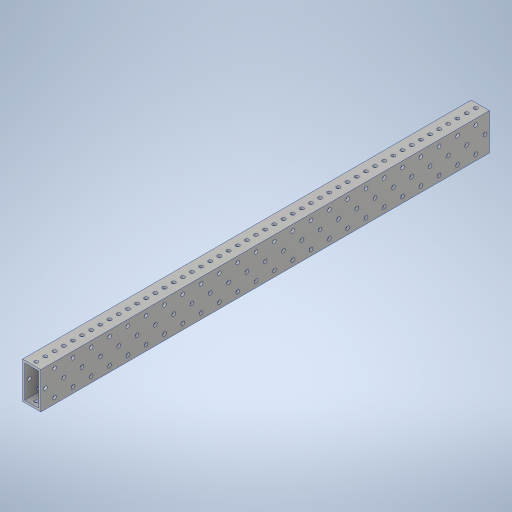
# Autodesk Inventor part: DB1-002
Saved by Autodesk Inventor 2023.4 (Build 274418000, 418)
## iProperties
Created: 2025-01-09
Part Number: DB1-002
Material: Aluminum 6061
Document SubType Name: Modeling
Designer: mavericks
Mass: 304.185 g
Surface Area: 718.547 cm^2
Volume: 112.661 cm^3
Density: 2.7 g/cm^3
Appearance: Aluminum - Flat
RuleStatus: InUse
AfterDocNew0: SHOW
AfterDocOpen0: SHOW
Author: mavericks
Autodesk Inventor part; units mm, degrees
ref_plane "YZ Plane" through (0, 0, 0) normal (1, 0, 0) x (0, 1, 0)
ref_plane "XZ Plane" through (0, 0, 0) normal (0, 1, 0) x (-1, 0, 0)
ref_plane "XY Plane" through (0, 0, 0) normal (0, 0, 1) x (1, 0, 0)
sketch "Sketch1" plane through (0, 0, 0) normal (0, 0, 1) x (1, 0, 0)
  line L0 (-12.7, -25.4) -> (12.7, -25.4)
  line L1 (12.7, -25.4) -> (12.7, 25.4)
  line L2 (12.7, 25.4) -> (-12.7, 25.4)
  line L3 (-12.7, 25.4) -> (-12.7, -25.4)
  line L4 (-12.7, -25.4) -> (12.7, 25.4) construction
  line L5 (12.7, -25.4) -> (-12.7, 25.4) construction
  line L6 (-9.525, 22.225) -> (9.525, 22.225)
  line L7 (9.525, 22.225) -> (9.525, -22.225)
  line L8 (9.525, -22.225) -> (-9.525, -22.225)
  line L9 (-9.525, -22.225) -> (-9.525, 22.225)
  point P0 (0, 0)
  dimension "width" = 25.4
  dimension "height" = 50.8
  dimension "thickness" = 3.175
  constraints: 20 end point, 4 parallel, 2 midpoint, 2 perpendicular, 1 horizontal, 3 other
  measures "width" distance of L2.end L1.end
  measures "height" distance of L1.end L0.end
  measures "thickness" distance between parallel lines of L2 L6
extrude "Extrusion1" add sketch "Sketch1" along normal mid plane 622.3
sketch "Sketch2" plane through (-12.7, 25.4, 311.15) normal (0, 1, 0) x (1, 0, 0)
  line L0 (12.7, 323.85) -> (12.7, 298.45) construction
  line L1 (0, 622.3) -> (0, 0) construction
  point P0 (12.7, 311.15)
  point P1 (12.7, 311.15)
  point P2 (12.7, 285.75)
  point P3 (12.7, 273.05)
  point P4 (12.7, 260.35)
  point P5 (12.7, 247.65)
  point P6 (12.7, 234.95)
  point P7 (12.7, 222.25)
  point P8 (12.7, 209.55)
  point P9 (12.7, 196.85)
  point P10 (12.7, 184.15)
  point P11 (12.7, 171.45)
  point P12 (12.7, 158.75)
  point P13 (12.7, 146.05)
  point P14 (12.7, 133.35)
  point P15 (12.7, 120.65)
  point P16 (12.7, 107.95)
  point P17 (12.7, 95.25)
  point P18 (12.7, 82.55)
  point P19 (12.7, 69.85)
  point P20 (12.7, 57.15)
  point P21 (12.7, 44.45)
  point P22 (12.7, 31.75)
  point P23 (12.7, 19.05)
  point P24 (12.7, 6.35)
  point P25 (12.7, 336.55)
  point P26 (12.7, 349.25)
  point P27 (12.7, 361.95)
  point P28 (12.7, 374.65)
  point P29 (12.7, 387.35)
  point P30 (12.7, 400.05)
  point P31 (12.7, 412.75)
  point P32 (12.7, 425.45)
  point P33 (12.7, 438.15)
  point P34 (12.7, 450.85)
  point P35 (12.7, 463.55)
  point P36 (12.7, 476.25)
  point P37 (12.7, 488.95)
  point P38 (12.7, 501.65)
  point P39 (12.7, 514.35)
  point P40 (12.7, 527.05)
  point P41 (12.7, 539.75)
  point P42 (12.7, 552.45)
  point P43 (12.7, 565.15)
  point P44 (12.7, 577.85)
  point P45 (12.7, 590.55)
  point P46 (12.7, 603.25)
  point P47 (12.7, 615.95)
  point P48 (12.7, 311.15)
  dimension "d6" = 25.4
  dimension "d9" = 12.7
  dimension "d16" = 12.7
  constraints: 3 vertical, 2 coincident, 2 end point, 2 vertical alignment, 1 midpoint, 46 other
  measures "d6" distance of L0.start L0.end
  measures "d9" distance of L0.end point (12.7, 285.75)
  measures "d16" distance of L0.start point (12.7, 336.55)
hole "Hole1" at (0, 25.4, 12.7) at (0, 25.4, -12.7) at (0, 25.4, 25.4) at (0, 25.4, 38.1) at (0, 25.4, 50.8) at (0, 25.4, 63.5) at (0, 25.4, 76.2) at (0, 25.4, 88.9) at (0, 25.4, 101.6) at (0, 25.4, 114.3) at (0, 25.4, 127) at (0, 25.4, 139.7) at (0, 25.4, 152.4) at (0, 25.4, 165.1) at (0, 25.4, 177.8) at (0, 25.4, 190.5) at (0, 25.4, 203.2) at (0, 25.4, 215.9) at (0, 25.4, 228.6) at (0, 25.4, 241.3) at (0, 25.4, 254) at (0, 25.4, 266.7) at (0, 25.4, 279.4) at (0, 25.4, 292.1) at (0, 25.4, 304.8) at (0, 25.4, -25.4) at (0, 25.4, -38.1) at (0, 25.4, -50.8) at (0, 25.4, -63.5) at (0, 25.4, -76.2) at (0, 25.4, -88.9) at (0, 25.4, -101.6) at (0, 25.4, -114.3) at (0, 25.4, -127) at (0, 25.4, -139.7) at (0, 25.4, -152.4) at (0, 25.4, -165.1) at (0, 25.4, -177.8) at (0, 25.4, -190.5) at (0, 25.4, -203.2) at (0, 25.4, -215.9) at (0, 25.4, -228.6) at (0, 25.4, -241.3) at (0, 25.4, -254) at (0, 25.4, -266.7) at (0, 25.4, -279.4) at (0, 25.4, -292.1) at (0, 25.4, -304.8) at (0, 25.4, 0) direction (0, -1, 0) diameter 5.1054 end through all clearance for "Flat Head Machine Screw (82)" size "#10" standard "Ansi Unified Screw Threads"
sketch "Sketch3" plane through (12.7, -25.4, 311.15) normal (1, 0, 0) x (0, 0, -1)
  line L0 (298.45, 42.8625) -> (298.45, 7.9375) construction
  circle A0 centre (298.45, 42.8625) radius 4.7625 construction
  line L1 (0, 47.625) -> (622.3, 47.625) construction
  circle A1 centre (298.45, 7.9375) radius 4.7625 construction
  line L2 (0, 3.175) -> (622.3, 3.175) construction
  line L3 (298.45, 42.8625) -> (323.85, 42.8625) construction
  point P0 (311.15, 25.4)
  point P1 (311.15, 25.4)
  point P2 (323.85, 7.9375)
  point P3 (273.05, 42.8625)
  point P4 (285.75, 25.4)
  point P5 (273.05, 7.9375)
  point P6 (247.65, 42.8625)
  point P7 (260.35, 25.4)
  point P8 (247.65, 7.9375)
  point P9 (222.25, 42.8625)
  point P10 (234.95, 25.4)
  point P11 (222.25, 7.9375)
  point P12 (196.85, 42.8625)
  point P13 (209.55, 25.4)
  point P14 (196.85, 7.9375)
  point P15 (171.45, 42.8625)
  point P16 (184.15, 25.4)
  point P17 (171.45, 7.9375)
  point P18 (146.05, 42.8625)
  point P19 (158.75, 25.4)
  point P20 (146.05, 7.9375)
  point P21 (120.65, 42.8625)
  point P22 (133.35, 25.4)
  point P23 (120.65, 7.9375)
  point P24 (95.25, 42.8625)
  point P25 (107.95, 25.4)
  point P26 (95.25, 7.9375)
  point P27 (69.85, 42.8625)
  point P28 (82.55, 25.4)
  point P29 (69.85, 7.9375)
  point P30 (44.45, 42.8625)
  point P31 (57.15, 25.4)
  point P32 (44.45, 7.9375)
  point P33 (19.05, 42.8625)
  point P34 (31.75, 25.4)
  point P35 (19.05, 7.9375)
  point P36 (-6.35, 42.8625)
  point P37 (6.35, 25.4)
  point P38 (-6.35, 7.9375)
  point P39 (336.55, 25.4)
  point P40 (336.55, 25.4)
  point P41 (349.25, 42.8625)
  point P42 (349.25, 7.9375)
  point P43 (361.95, 25.4)
  point P44 (361.95, 25.4)
  point P45 (374.65, 42.8625)
  point P46 (374.65, 7.9375)
  point P47 (387.35, 25.4)
  point P48 (387.35, 25.4)
  point P49 (400.05, 42.8625)
  point P50 (400.05, 7.9375)
  point P51 (412.75, 25.4)
  point P52 (412.75, 25.4)
  point P53 (425.45, 42.8625)
  point P54 (425.45, 7.9375)
  point P55 (438.15, 25.4)
  point P56 (438.15, 25.4)
  point P57 (450.85, 42.8625)
  point P58 (450.85, 7.9375)
  point P59 (463.55, 25.4)
  point P60 (463.55, 25.4)
  point P61 (476.25, 42.8625)
  point P62 (476.25, 7.9375)
  point P63 (488.95, 25.4)
  point P64 (488.95, 25.4)
  point P65 (501.65, 42.8625)
  point P66 (501.65, 7.9375)
  point P67 (514.35, 25.4)
  point P68 (514.35, 25.4)
  point P69 (527.05, 42.8625)
  point P70 (527.05, 7.9375)
  point P71 (539.75, 25.4)
  point P72 (539.75, 25.4)
  point P73 (552.45, 42.8625)
  point P74 (552.45, 7.9375)
  point P75 (565.15, 25.4)
  point P76 (565.15, 25.4)
  point P77 (577.85, 42.8625)
  point P78 (577.85, 7.9375)
  point P79 (590.55, 25.4)
  point P80 (590.55, 25.4)
  point P81 (603.25, 42.8625)
  point P82 (603.25, 7.9375)
  point P83 (615.95, 25.4)
  point P84 (615.95, 25.4)
  point P85 (628.65, 42.8625)
  point P86 (628.65, 7.9375)
  dimension "d28" = 12.7
  dimension "d29" = 9.525
  dimension "d30" = 9.525
  dimension "d31" = 25.4
  dimension "d34" = 25.4
  dimension "d41" = 25.4
  constraints: 17 coincident, 4 end point, 3 horizontal, 2 centre point, 2 horizontal alignment, 2 tangent, 2 vertical alignment, 1 vertical, 84 other
  measures "d28" horizontal distance of point (311.15, 25.4) L0.start
  measures "d29" diameter of A0
  measures "d30" diameter of A1
  measures "d31" distance of L3.end L3.start
  measures "d34" distance of L0.start point (273.05, 42.863)
  measures "d41" distance of point (311.15, 25.4) point (336.55, 25.4)
hole "Hole2" at (12.7, 0, 0) at (12.7, 17.4625, 12.7) at (12.7, 17.4625, -12.7) at (12.7, -17.4625, -12.7) at (12.7, -17.4625, 12.7) at (12.7, 17.4625, 38.1) at (12.7, 0, 25.4) at (12.7, -17.4625, 38.1) at (12.7, 17.4625, 63.5) at (12.7, 0, 50.8) at (12.7, -17.4625, 63.5) at (12.7, 17.4625, 88.9) at (12.7, 0, 76.2) at (12.7, -17.4625, 88.9) at (12.7, 17.4625, 114.3) at (12.7, 0, 101.6) at (12.7, -17.4625, 114.3) at (12.7, 17.4625, 139.7) at (12.7, 0, 127) at (12.7, -17.4625, 139.7) at (12.7, 17.4625, 165.1) at (12.7, 0, 152.4) at (12.7, -17.4625, 165.1) at (12.7, 17.4625, 190.5) at (12.7, 0, 177.8) at (12.7, -17.4625, 190.5) at (12.7, 17.4625, 215.9) at (12.7, 0, 203.2) at (12.7, -17.4625, 215.9) at (12.7, 17.4625, 241.3) at (12.7, 0, 228.6) at (12.7, -17.4625, 241.3) at (12.7, 17.4625, 266.7) at (12.7, 0, 254) at (12.7, -17.4625, 266.7) at (12.7, 17.4625, 292.1) at (12.7, 0, 279.4) at (12.7, -17.4625, 292.1) at (12.7, 17.4625, 317.5) at (12.7, 0, 304.8) at (12.7, -17.4625, 317.5) at (12.7, 0, -25.4) at (12.7, 17.4625, -38.1) at (12.7, -17.4625, -38.1) at (12.7, 0, -50.8) at (12.7, 17.4625, -63.5) at (12.7, -17.4625, -63.5) at (12.7, 0, -76.2) at (12.7, 17.4625, -88.9) at (12.7, -17.4625, -88.9) direction (-1, 0, 0) diameter 5.1054 end through all and at (12.7, 0, -101.6) (12.7, 17.4625, -114.3) (12.7, -17.4625, -114.3) (12.7, 0, -127) (12.7, 17.4625, -139.7) (12.7, -17.4625, -139.7) (12.7, 0, -152.4) (12.7, 17.4625, -165.1) (12.7, -17.4625, -165.1) (12.7, 0, -177.8) (12.7, 17.4625, -190.5) (12.7, -17.4625, -190.5) (12.7, 0, -203.2) (12.7, 17.4625, -215.9) (12.7, -17.4625, -215.9) (12.7, 0, -228.6) (12.7, 17.4625, -241.3) (12.7, -17.4625, -241.3) (12.7, 0, -254) (12.7, 17.4625, -266.7) (12.7, -17.4625, -266.7) (12.7, 0, -279.4) (12.7, 17.4625, -292.1) (12.7, -17.4625, -292.1) (12.7, 0, -304.8) (12.7, 17.4625, -317.5) (12.7, -17.4625, -317.5) clearance for "Flat Head Machine Screw (82)" size "#10" standard "Ansi Unified Screw Threads"
body "Solid1"
